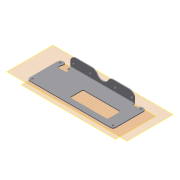
# Autodesk Inventor part: oled br
Saved by Autodesk Inventor 2014 (Build 180170000, 170)
## iProperties
Created: 2016-03-30
Part Number: oled br
Material: Generic
Document SubType Name: Sheet Metal
Designer: admin
Density: 1 g/cm^3
Sheet Metal Rule: Default_mm
Appearance: Default
Author: admin
Autodesk Inventor part; units mm, degrees
ref_plane "YZ Plane" through (0, 0, 0) normal (1, 0, 0) x (0, 1, 0)
ref_plane "XZ Plane" through (0, 0, 0) normal (0, 1, 0) x (-1, 0, 0)
ref_plane "XY Plane" through (0, 0, 0) normal (0, 0, 1) x (1, 0, 0)
ref_plane "Work Plane1" through (0, 0, 0) normal (0, 0, 1) x (1, 0, 0)
sketch "Sketch1" plane through (0, 0, 0) normal (0, 0, 1) x (1, 0, 0)
  circle A0 centre (-72.5, -8) radius 1.6
  circle A1 centre (-72.5, -58) radius 1.6
  circle A2 centre (72.5, -58) radius 1.6
  circle A3 centre (72.5, -8) radius 1.6
  line L0 (17.5, 3) -> (17.5, -3)
  line L1 (-17.5, 3) -> (17.5, 3)
  line L2 (-17.5, -3) -> (-17.5, 3)
  line L3 (-77.5, -3) -> (-17.5, -3)
  line L4 (-77.5, -63) -> (-77.5, -3)
  line L5 (77.5, -63) -> (-77.5, -63)
  line L6 (77.5, -3) -> (77.5, -63)
  line L7 (17.5, -3) -> (77.5, -3)
  line L8 (-5.5, -46) -> (-5.5, -36)
  line L9 (19.5, -46) -> (-5.5, -46)
  line L10 (19.5, -36) -> (19.5, -46)
  line L11 (-5.5, -36) -> (19.5, -36)
  line L12 (-4.5, -45) -> (-4.5, -37)
  line L13 (-4.5, -37) -> (18.5, -37)
  line L14 (18.5, -37) -> (18.5, -45)
  line L15 (18.5, -45) -> (-4.5, -45)
  line L16 (33.5, -45) -> (33.5, -37)
  line L17 (33.5, -37) -> (51.5, -37)
  line L18 (51.5, -37) -> (51.5, -45)
  line L19 (51.5, -45) -> (33.5, -45)
  line L20 (32.5, -46) -> (32.5, -36)
  line L21 (52.5, -46) -> (32.5, -46)
  line L22 (52.5, -36) -> (52.5, -46)
  line L23 (32.5, -36) -> (52.5, -36)
  line L24 (-54, -11) -> (-67.5, -11)
  line L25 (-67.5, -11) -> (-67.5, -16)
  line L26 (-67.5, -16) -> (-55.5, -16)
  line L27 (-55.5, -16) -> (-54, -14.5)
  line L28 (-54, -14.5) -> (-54, -11)
  line L29 (-53, -17) -> (-68.5, -17)
  line L30 (-68.5, -17) -> (-68.5, -10)
  line L31 (-68.5, -10) -> (-53, -10)
  line L32 (-53, -10) -> (-53, -17)
  line L33 (-10.5, -29) -> (57.5, -29)
  line L34 (57.5, -29) -> (57.5, -53)
  line L35 (57.5, -53) -> (-10.5, -53)
  line L36 (-10.5, -53) -> (-10.5, -29)
  line L37 (-17.5, -3) -> (17.5, -3)
  point P0 (0, 0)
  dimension "d0" = 1
  dimension "d1" = 1
  dimension "d2" = 1
  dimension "d3" = 1
  dimension "d4" = 5
  dimension "d5" = 7
  dimension "d6" = 5
  dimension "d7" = 7
  measures "d0" distance between parallel lines of L31 L24
  measures "d1" distance between parallel lines of L29 L26
  measures "d2" distance between parallel lines of L32 L28
  measures "d3" distance between parallel lines of L25 L30
  measures "d4" distance between parallel lines of L8 L36
  measures "d5" distance between parallel lines of L33 L11
  measures "d6" distance between parallel lines of L34 L22
  measures "d7" distance between parallel lines of L35 L21
extrude "Plate1" add sketch "Sketch1" along normal blind 1.5 contours L7 L6 L5 L4 L3 L37
fillet "Fillet1" radius 1 4 edges at (-53, -10, 0.75) (-68.5, -10, 0.75) (-68.5, -17, 0.75) (-53, -17, 0.75)
ref_plane "Work Plane2" through (0, 0, -10) normal (0, 0, 1) x (1, 0, 0)
sketch "Sketch7" plane through (0, 0, 1.5) normal (0, 0, 1) x (1, 0, 0)
  line L0 (-67.5, -10) -> (-54, -10) projected
  circle A0 centre (-72.5, -8) radius 1.6 projected
  line L1 (-77.5, -3) -> (77.5, -3) projected
  line L2 (-77.5, -63) -> (-77.5, -3) projected
  line L3 (77.5, -3) -> (77.5, -63) projected
  line L4 (-67.5, -3) -> (-67.5, -10)
  line L5 (-57.5, -3) -> (-57.5, -10)
  line L6 (67.5, -3) -> (67.5, -8)
  line L7 (57.5, -3) -> (57.5, -8)
  line L8 (57.5, -8) -> (67.5, -8)
  line L9 (-77.5, -3.1) -> (77.5, -3.1)
  point P0 (0, 0)
  dimension "d49" = 5
  dimension "d50" = 10
  dimension "d51" = 10
  dimension "d52" = 10
  dimension "d53" = 5
  dimension "d54" = 0.1
  constraints: 12 end point, 8 point on line, 3 parallel, 3 perpendicular
  measures "d49" distance from line of A0.centre L4
  measures "d50" distance between parallel lines of L4 L5
  measures "d51" distance between parallel lines of L3 L6
  measures "d52" distance between parallel lines of L7 L6
  measures "d53" distance between parallel lines of L1 L8
  measures "d54" distance between parallel lines of L1 L9
extrude "Extrusion4" cut sketch "Sketch7" against normal blind 2 contours L4 L9 L5 L0 | L9 L2 L1 L4 | L4 L1 L5 L9 | L5 L1 L7 L9 | L9 L6 L8 L7 | L7 L1 L6 L9 | L6 L1 L3 L9
sketch "Sketch8" plane through (-57.5, -4.5991, -0.0523) normal (0, 0.9993908, 0.0348995) x (-1, 0, 0)
  line L0 (-115, 0) -> (0, 0)
  line L1 (0, 0) -> (0, 20)
  line L2 (0, 20) -> (-115, 20)
  line L3 (-115, 20) -> (-115, 0)
  constraints: 6 end point, 1 horizontal, 1 perpendicular, 1 vertical
edge flange "Flange3" height 20 angle 92 thickness 1.5 bend radius 1.5 thickness toward (0, 0.9993908, 0.0348995) relief tear relief width 1.5 relief depth 0.75 edges at (0, -3.1, 1.5) wall of the first edge with corners at (57.5, -4.5991, -0.0523) (-57.5, -4.5991, -0.0523) (-57.5, -5.2971, 19.9355) (57.5, -5.2971, 19.9355)
bend "Bend3"
corner "Corner3"
fillet "Fillet2" radius 5 4 edges at (-77.5, -3.1, 0.75) (-77.5, -63, 0.75) (77.5, -63, 0.75) (77.5, -3.1, 0.75)
fillet "Fillet3" radius 2 2 edges at (67.5, -3.1, 0.75) (-67.5, -3.1, 0.75)
sketch "Sketch9" plane through (-57.5, -5.2971, 19.9355) normal (0, -0.9993908, -0.0348995) x (1, 0, 0)
  line L0 (115, 0) -> (115, -16.8934) projected
  line L1 (115, 0) -> (0, 0) projected
  line L2 (0, 0) -> (0, -16.8934) projected
  circle A0 centre (5, -11) radius 1.5
  circle A1 centre (35, -11) radius 1.5
  circle A2 centre (80, -11) radius 1.5
  circle A3 centre (110, -11) radius 1.5
  point P0 (57.5, -20.1082)
  dimension "d69" = 3
  dimension "d70" = 3
  dimension "d71" = 3
  dimension "d72" = 3
  dimension "d73" = 5
  dimension "d74" = 5
  dimension "d75" = 30
  dimension "d76" = 30
  dimension "d77" = 11
  dimension "d78" = 11
  dimension "d79" = 11
  dimension "d80" = 11
  constraints: 4 centre point
  measures "d69" diameter of A0
  measures "d70" diameter of A1
  measures "d71" diameter of A2
  measures "d72" diameter of A3
  measures "d73" distance from line of L2 A0.centre
  measures "d74" distance from line of L0 A3.centre
  measures "d75" distance of A1.centre A0.centre
  measures "d76" distance of A3.centre A2.centre
  measures "d77" distance from line of L1 A0.centre
  measures "d78" distance from line of L1 A1.centre
  measures "d79" distance from line of L1 A2.centre
  measures "d80" distance from line of L1 A3.centre
extrude "Extrusion5" cut sketch "Sketch9" against normal blind 2
fillet "Fillet4" radius 10 2 edges at (57.5, -4.5475, 19.9616) (-57.5, -4.5475, 19.9616)
fillet "Fillet5" radius 2 4 edges at (-10.5, -29, 0.75) (-10.5, -53, 0.75) (57.5, -29, 0.75) (57.5, -53, 0.75)
sketch "Sketch10" plane through (-57.5, -4.7075, 3.0523) normal (0, -0.9993908, -0.0348995) x (1, 0, 0)
  line L0 (0, 0) -> (115, 0) projected
  line L1 (105, 16.8934) -> (10, 16.8934) projected
  circle A0 centre (57.5, 16.8934) radius 11.8934
  line L2 (57.5, 0) -> (57.5, 5)
  point P0 (57.5, -3.2148)
  dimension "d85" = 5
  constraints: 2 end point, 2 midpoint, 1 perpendicular, 1 vertical alignment, 2 other
  measures "d85" distance of L2.start L2.end
extrude "Extrusion6" cut sketch "Sketch10" against normal blind 10
fillet "Fillet6" radius 10 2 edges at (-11.8934, -4.5475, 19.9616) (11.8934, -4.5475, 19.9616)
equation "\"d57\" = BendReliefWidth"
equation "\"d58\" = BendReliefDepth"
equation "\"d59\" = MinimumRemnant"
equation "\"d60\" = BendRadius"
equation "\"d63\" = BendRadius"
equation "\"d64\" = CornerReliefSize"
equation "\"d65\" = GapSize"
equation "\"d66\" = JacobiRadiusSize"
equation "\"BendRadius\" = Thickness"
equation "\"BendReliefWidth\" = Thickness"
equation "\"BendReliefDepth\" = 0.5 * Thickness"
equation "\"CornerReliefSize\" = 4 * Thickness"
equation "\"MinimumRemnant\" = 2 * Thickness"
equation "\"TransitionRadius\" = BendRadius"
equation "\"JacobiRadiusSize\" = BendRadius"
equation "\"GapSize\" = Thickness"
equation "\"d8\" = BendRadius"
equation "\"Thickness\" = 1.5"
body "Solid1"
